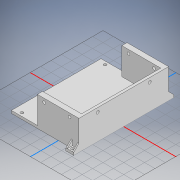
# Autodesk Inventor part: 000.003.001 - Основание
Saved by Autodesk Inventor 2022 (Build 260153000, 153)
## iProperties
Created: 2022-02-26
Part Number: 000.003.001 - Основание
Material: Типовые
Document SubType Name: Modeling
Designer: Petrov Ivan
Density: 1 g/cm^3
Appearance: По умолчанию
Author: Petrov Ivan
Autodesk Inventor part; units mm, degrees
ref_plane "YZ Plane" through (0, 0, 0) normal (1, 0, 0) x (0, 1, 0)
ref_plane "XZ Plane" through (0, 0, 0) normal (0, 1, 0) x (-1, 0, 0)
ref_plane "XY Plane" through (0, 0, 0) normal (0, 0, 1) x (1, 0, 0)
sketch "Эскиз1" plane through (0, 0, 0) normal (0, 1, 0) x (-1, 0, 0)
  line L0 (40, 86.25) -> (-40, 86.25)
  line L1 (-40, 86.25) -> (-40, -86.25)
  line L2 (-40, -86.25) -> (40, -86.25)
  line L3 (40, -86.25) -> (40, 86.25)
  point P0 (0, 0)
  dimension "d0" = 80
  dimension "d1" = 172.5
  dimension "d29" = 86.25
  dimension "d30" = 40
  constraints: 8 end point, 2 parallel, 1 horizontal, 1 perpendicular
  measures "d0" distance of L2.end L1.end
  measures "d1" distance of L1.end L0.end
  measures "d29" distance from line of point (0, 0) L2
  measures "d30" distance from line of point (0, 0) L1
extrude "Выдавливание1" add sketch "Эскиз1" along normal blind 5
sketch "Эскиз3" plane through (0, 5, 0) normal (0, 1, 0) x (1, 0, 0)
  line L0 (-40, 86.25) -> (-40, -86.25) projected
  line L1 (-40, 86.25) -> (-40, 76.25)
  line L2 (-40, 76.25) -> (35, 76.25)
  line L3 (35, 76.25) -> (35, -76.25)
  line L4 (35, -76.25) -> (-40, -76.25)
  line L5 (-40, -86.25) -> (40, -86.25) projected
  line L6 (40, 86.25) -> (-40, 86.25) projected
  line L7 (40, -86.25) -> (40, 86.25) projected
  point P0 (0, 0)
  point P1 (-40, -76.25)
  dimension "d11" = 10
  dimension "d12" = 10
  dimension "d13" = 5
  constraints: 8 end point, 2 perpendicular, 2 point on line, 1 horizontal
  measures "d11" distance between parallel lines of L4 L5
  measures "d12" distance between parallel lines of L6 L2
  measures "d13" distance between parallel lines of L7 L3
extrude "Выдавливание3" add sketch "Эскиз3" along normal blind 51.75 contours L6 L7 L5 L0 L4 L3 L2
sketch "Эскиз4" plane through (0, 0, 0) normal (0, -1, 0) x (1, 0, 0)
  line L0 (-40, 86.25) -> (40, 86.25) projected
  line L1 (40, 86.25) -> (25, 86.25)
  line L2 (25, 86.25) -> (25, 96.25)
  line L3 (25, 96.25) -> (40, 96.25)
  line L4 (40, 96.25) -> (40, 86.25)
  circle A0 centre (32.5, 91.25) radius 2.775
  point P0 (0, 0)
  point P1 (32.5, 96.25)
  dimension "d16" = 15
  dimension "d17" = 10
  dimension "d18" = 5.55
  constraints: 8 end point, 2 parallel, 1 centre point, 1 horizontal, 1 midpoint, 1 perpendicular, 1 vertical alignment
  measures "d16" distance of L2.end L3.end
  measures "d17" distance of L1.end L2.end
  measures "d18" diameter of A0
extrude "Выдавливание4" add sketch "Эскиз4" against normal blind 5
sketch "Эскиз5" plane through (0, 5, 0) normal (0, 1, 0) x (1, 0, 0)
  line L0 (25, -86.25) -> (25, -96.25) projected
  line L1 (-40, -86.25) -> (40, -86.25) projected
  line L2 (25, -96.25) -> (27.5, -96.25)
  line L3 (27.5, -96.25) -> (27.5, -86.25)
  line L4 (27.5, -86.25) -> (25, -86.25)
  line L5 (25, -86.25) -> (25, -96.25)
  line L6 (40, -96.25) -> (40, 86.25) projected
  line L7 (40, -96.25) -> (37.5, -96.25)
  line L8 (37.5, -96.25) -> (37.5, -86.25)
  line L9 (37.5, -86.25) -> (40, -86.25)
  line L10 (40, -86.25) -> (40, -96.25)
  point P0 (0, 0)
  dimension "d21" = 2.5
  dimension "d22" = 2.5
  constraints: 16 end point, 4 parallel, 2 horizontal, 2 perpendicular, 2 point on line
  measures "d21" distance between parallel lines of L0 L3
  measures "d22" distance between parallel lines of L6 L8
extrude "Выдавливание5" add sketch "Эскиз5" along normal blind 10
chamfer "Фаска1" distance 10 angle 45 2 edges at (26.25, 15, 96.25) (38.75, 15, 96.25)
mirror "Зеркальное отражение3" about plane through (0, 0, 0) normal (0, 0, 1) of "Выдавливание4", "Выдавливание5", "Фаска1"
sketch "Эскиз6" plane through (-40, 0, -86.25) normal (-1, 0, 0) x (0, 0, 1)
  line L0 (172.5, 0) -> (172.5, 15) projected
  line L1 (0, 0) -> (0, 56.75) projected
  line L2 (172.5, 5) -> (0, 5)
  line L3 (0, 5) -> (0, 0)
  line L4 (0, 0) -> (172.5, 0)
  line L5 (172.5, 0) -> (172.5, 5)
  point P0 (86.25, 0)
  point P1 (10, 5)
  point P2 (0, 5)
  constraints: 8 end point, 2 parallel, 2 point on line, 1 horizontal, 1 perpendicular
extrude "Выдавливание6" add sketch "Эскиз6" along normal blind 50
sketch "Эскиз7" plane through (0, 5, 0) normal (0, 1, 0) x (1, 0, 0)
  circle A0 centre (-76, 80) radius 4 projected
  circle A1 centre (-76, -80) radius 4 projected
  circle A2 centre (-76, 80) radius 2.75
  circle A3 centre (-76, -80) radius 2.75
  point P0 (0, 0)
  dimension "d33" = 5.5
  dimension "d34" = 5.5
  constraints: 2 centre point, 2 coincident
  measures "d33" diameter of A2
  measures "d34" diameter of A3
extrude "Выдавливание7" cut sketch "Эскиз7" against normal through all contours A2 | A3
sketch "Эскиз8" plane through (-40, 56.75, 86.25) normal (0, 0, 1) x (1, 0, 0)
  circle A0 centre (13, -7) radius 2.75
  circle A1 centre (62, -7) radius 2.75
  line L0 (75, -51.75) -> (75, 0) projected
  line L1 (77.5, -41.75) -> (80, -41.75) projected
  line L2 (80, -41.75) -> (80, 0) projected
  line L3 (0, 0) -> (80, 0) projected
  line L4 (0, -51.75) -> (0, 0) projected
  line L5 (0, -51.75) -> (-50, -51.75) projected
  line L6 (-50, -56.75) -> (-50, -51.75) projected
  line L7 (65, -56.75) -> (-50, -56.75) projected
  line L8 (65, -56.75) -> (65, -41.75) projected
  line L9 (65, -41.75) -> (67.5, -41.75) projected
  line L10 (67.5, -41.75) -> (67.5, -51.75) projected
  line L11 (67.5, -51.75) -> (77.5, -51.75) projected
  line L12 (77.5, -51.75) -> (77.5, -41.75) projected
  point P0 (40, -56.75)
  dimension "d37" = 5.5
  dimension "d38" = 5.5
  dimension "d39" = 7
  dimension "d40" = 13
  dimension "d41" = 13
  constraints: 2 centre point, 1 horizontal alignment
  measures "d37" diameter of A0
  measures "d38" diameter of A1
  measures "d39" distance from line of L3 A1.centre
  measures "d40" distance from line of L0 A1.centre
  measures "d41" distance from line of L4 A0.centre
extrude "Выдавливание8" cut sketch "Эскиз8" against normal through all contours A0 | A1
sketch "Эскиз9" plane through (40, 56.75, 86.25) normal (1, 0, 0) x (0, 0, -1)
  circle A0 centre (36.25, -8) radius 2.75
  circle A1 centre (136.25, -8) radius 2.75
  line L0 (0, 0) -> (172.5, 0) projected
  line L1 (162.5, 0) -> (10, 0) projected
  line L2 (86.25, 0) -> (86.25, -11.5719) construction
  point P0 (86.25, -56.75)
  dimension "d44" = 5.5
  dimension "d45" = 5.5
  dimension "d46" = 8
  dimension "d50" = 50
  constraints: 2 centre point, 2 end point, 1 horizontal alignment, 1 midpoint, 1 symmetric about line, 1 vertical
  measures "d44" diameter of A0
  measures "d45" diameter of A1
  measures "d46" distance from line of L0 A0.centre
  measures "d50" distance from line of L2 A0.centre
extrude "Выдавливание9" cut sketch "Эскиз9" against normal blind 10
equation "\"d29\" = 0.5 * d1"
equation "\"d30\" = 0.5 * d0"
equation "\"d12\" = d11"
equation "\"d34\" = d33"
